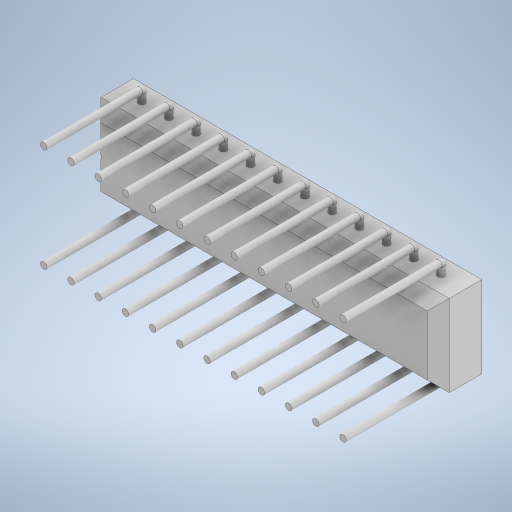
# Autodesk Inventor part: LM1040
Saved by Autodesk Inventor 2024 (Build 280153000, 153)
## iProperties
Created: 2023-12-15
Part Number: LM1040
Material: Generic
Document SubType Name: Sheet Metal
Designer: user
Density: 1 g/cm^3
Sheet Metal Rule: Default
Appearance: Default
Author: user
Autodesk Inventor part; units mm, degrees
sketch "Sketch1" plane through (0, 0, 0) normal (0, 0, 1) x (1, 0, 0)
  line L0 (0, 0) -> (32, 0)
  line L1 (32, 0) -> (32, 7.5)
  line L2 (32, 7.5) -> (0, 7.5)
  line L3 (0, 7.5) -> (0, 5)
  line L4 (0, 0) -> (0, 2.5)
  arc A0 (0, 2.5) -> (0, 5) centre (-0.2534, 3.75) ccw
  dimension "d0" = 32
  dimension "d1" = 7.5
  dimension "d2" = 2.5
  dimension "d3" = 2.5
  constraints: 10 end point, 2 point on circle, 2 vertical, 1 centre point, 1 horizontal, 1 parallel, 1 perpendicular
  measures "d0" distance of L2.end L1.end
  measures "d1" distance of L1.end L0.end
  measures "d2" distance of L2.end L3.end
  measures "d3" distance of L0.start L4.end
extrude "Extrusion1" add sketch "Sketch1" along normal blind 5
sketch "Sketch2" plane through (0, 7.5, 0) normal (0, 1, 0) x (1, 0, 0)
  line L0 (0, 0) -> (0, -5) projected
  circle A0 centre (29.75, -2.5) radius 0.3
  circle A1 centre (27.25, -2.5) radius 0.3
  circle A2 centre (24.75, -2.5) radius 0.3
  circle A3 centre (22.25, -2.5) radius 0.3
  circle A4 centre (19.75, -2.5) radius 0.3
  circle A5 centre (17.25, -2.5) radius 0.3
  circle A6 centre (14.75, -2.5) radius 0.3
  circle A7 centre (12.25, -2.5) radius 0.3
  circle A8 centre (9.75, -2.5) radius 0.3
  circle A9 centre (7.25, -2.5) radius 0.3
  circle A10 centre (4.75, -2.5) radius 0.3
  circle A11 centre (2.25, -2.5) radius 0.3
  line L1 (32, 0) -> (32, -5) projected
  line L2 (32, -2.5) -> (31.5682, -2.5)
  line L3 (0, -5) -> (32, -5) projected
  line L4 (32, -5) -> (29.75, -5)
  line L5 (29.75, -5) -> (27.25, -5)
  line L6 (27.25, -5) -> (24.75, -5)
  line L7 (24.75, -5) -> (22.25, -5)
  line L8 (22.25, -5) -> (19.75, -5)
  line L9 (19.75, -5) -> (17.25, -5)
  line L10 (17.25, -5) -> (14.75, -5)
  line L11 (14.75, -5) -> (12.25, -5)
  line L12 (12.25, -5) -> (9.75, -5)
  line L13 (9.75, -5) -> (7.25, -5)
  line L14 (7.25, -5) -> (4.75, -5)
  line L15 (4.75, -5) -> (2.25, -5)
  dimension "d8" = 0.6
  dimension "d10" = 0.6
  dimension "d21" = 0.6
  dimension "d22" = 0.6
  dimension "d23" = 0.6
  dimension "d24" = 0.6
  dimension "d25" = 0.6
  dimension "d26" = 0.6
  dimension "d27" = 0.6
  dimension "d28" = 0.6
  dimension "d29" = 0.6
  dimension "d30" = 0.6
  constraints: 26 end point, 12 centre point, 1 midpoint, 13 other
  measures "d8" diameter of A0
  measures "d10" diameter of A1
  measures "d21" diameter of A2
  measures "d22" diameter of A3
  measures "d23" diameter of A4
  measures "d24" diameter of A5
  measures "d25" diameter of A6
  measures "d26" diameter of A7
  measures "d27" diameter of A8
  measures "d28" diameter of A9
  measures "d29" diameter of A10
  measures "d30" diameter of A11
ref_plane "Work Plane1" through (29.75, 7.5, 5) normal (-1, 0, 0) x (0, -1, 0)
ref_plane "Work Plane2" through (27.25, 7.5, 5) normal (-1, 0, 0) x (0, -1, 0)
ref_plane "Work Plane3" through (24.75, 7.5, 5) normal (-1, 0, 0) x (0, -1, 0)
ref_plane "Work Plane4" through (22.25, 7.5, 5) normal (-1, 0, 0) x (0, -1, 0)
ref_plane "Work Plane5" through (19.75, 7.5, 5) normal (-1, 0, 0) x (0, -1, 0)
ref_plane "Work Plane6" through (17.25, 7.5, 5) normal (-1, 0, 0) x (0, -1, 0)
ref_plane "Work Plane7" through (14.75, 7.5, 5) normal (-1, 0, 0) x (0, -1, 0)
ref_plane "Work Plane8" through (12.25, 7.5, 5) normal (-1, 0, 0) x (0, -1, 0)
ref_plane "Work Plane9" through (9.75, 7.5, 5) normal (-1, 0, 0) x (0, -1, 0)
ref_plane "Work Plane10" through (7.25, 7.5, 5) normal (-1, 0, 0) x (0, -1, 0)
ref_plane "Work Plane11" through (4.75, 7.5, 5) normal (-1, 0, 0) x (0, -1, 0)
ref_plane "Work Plane12" through (2.25, 7.5, 5) normal (-1, 0, 0) x (0, -1, 0)
sketch "Sketch3" plane through (29.75, 7.5, 5) normal (-1, 0, 0) x (0, -1, 0)
  line L0 (0, -2.5) -> (-0.8, -2.5)
  line L1 (-1, -2.3) -> (-1, 6.5)
  arc A0 (-1, -2.3) -> (-0.8, -2.5) centre (-0.8, -2.3) ccw
  line L2 (0, -2.5) -> (7.5, -2.5)
  line L3 (7.5, -5) -> (7.5, 0) projected
  line L4 (7.5, -2.5) -> (8.3, -2.5)
  line L5 (8.5, -2.3) -> (8.5, 6.5)
  arc A1 (8.3, -2.5) -> (8.5, -2.3) centre (8.3, -2.3) ccw
  point P0 (0, -5)
  point P1 (-1, -2.5)
  point P2 (8.5, -2.5)
  dimension "d31" = 2.5
  dimension "d32" = 1
  dimension "d33" = 9
  dimension "d34" = 0.2
  dimension "d37" = 1
  dimension "d38" = 9
  dimension "d39" = 0.2
  constraints: 10 end point, 5 point on line, 4 point on circle, 4 tangent, 2 centre point, 2 perpendicular, 1 midpoint
  measures "d31" distance of point (0, -5) L0.start
  measures "d32" distance of L0.start point (-1, -2.5)
  measures "d33" distance of point (-1, -2.5) L1.end
  measures "d34" radius of A0
  measures "d37" distance of L2.end point (8.5, -2.5)
  measures "d38" distance of point (8.5, -2.5) L5.end
  measures "d39" radius of A1
sweep "Sweep1" add profiles "Sketch2" path "Sketch3" path curves L1 A0 L0 L2 L4 A1 L5 contours A0
sketch "Sketch4" plane through (27.25, 7.5, 5) normal (-1, 0, 0) x (0, -1, 0)
  line L0 (0, -2.5) -> (-0.8, -2.5)
  line L1 (-1, -2.3) -> (-1, 6.5)
  arc A0 (-1, -2.3) -> (-0.8, -2.5) centre (-0.8, -2.3) ccw
  line L2 (0, -2.5) -> (7.5, -2.5)
  line L3 (7.5, -2.5) -> (8.3, -2.5)
  line L4 (8.5, -2.3) -> (8.5, 6.5)
  arc A1 (8.3, -2.5) -> (8.5, -2.3) centre (8.3, -2.3) ccw
  point P0 (0, -5)
  point P1 (-1, -2.5)
  point P2 (8.5, -2.5)
  dimension "d40" = 2.5
  dimension "d41" = 1
  dimension "d42" = 9
  dimension "d43" = 0.2
  dimension "d44" = 1
  dimension "d45" = 9
  dimension "d46" = 0.2
  constraints: 10 end point, 5 point on line, 4 point on circle, 4 tangent, 2 centre point, 2 perpendicular
  measures "d40" distance of point (0, -5) L0.start
  measures "d41" distance of L0.start point (-1, -2.5)
  measures "d42" distance of point (-1, -2.5) L1.end
  measures "d43" radius of A0
  measures "d44" distance of L2.end point (8.5, -2.5)
  measures "d45" distance of point (8.5, -2.5) L4.end
  measures "d46" radius of A1
sketch "Sketch5" plane through (24.75, 7.5, 5) normal (-1, 0, 0) x (0, -1, 0)
  line L0 (0, -2.5) -> (-0.8, -2.5)
  line L1 (-1, -2.3) -> (-1, 6.5)
  arc A0 (-1, -2.3) -> (-0.8, -2.5) centre (-0.8, -2.3) ccw
  line L2 (0, -2.5) -> (7.5, -2.5)
  line L3 (7.5, -2.5) -> (8.3, -2.5)
  line L4 (8.5, -2.3) -> (8.5, 6.5)
  arc A1 (8.3, -2.5) -> (8.5, -2.3) centre (8.3, -2.3) ccw
  point P0 (0, -5)
  point P1 (-1, -2.5)
  point P2 (8.5, -2.5)
  dimension "d47" = 2.5
  dimension "d48" = 1
  dimension "d49" = 9
  dimension "d50" = 0.2
  dimension "d51" = 1
  dimension "d52" = 9
  dimension "d53" = 0.2
  constraints: 10 end point, 5 point on line, 4 point on circle, 4 tangent, 2 centre point, 2 perpendicular
  measures "d47" distance of point (0, -5) L0.start
  measures "d48" distance of L0.start point (-1, -2.5)
  measures "d49" distance of point (-1, -2.5) L1.end
  measures "d50" radius of A0
  measures "d51" distance of L2.end point (8.5, -2.5)
  measures "d52" distance of point (8.5, -2.5) L4.end
  measures "d53" radius of A1
sketch "Sketch6" plane through (22.25, 7.5, 5) normal (-1, 0, 0) x (0, -1, 0)
  line L0 (0, -2.5) -> (-0.8, -2.5)
  line L1 (-1, -2.3) -> (-1, 6.5)
  arc A0 (-1, -2.3) -> (-0.8, -2.5) centre (-0.8, -2.3) ccw
  line L2 (0, -2.5) -> (7.5, -2.5)
  line L3 (7.5, -2.5) -> (8.3, -2.5)
  line L4 (8.5, -2.3) -> (8.5, 6.5)
  arc A1 (8.3, -2.5) -> (8.5, -2.3) centre (8.3, -2.3) ccw
  point P0 (0, -5)
  point P1 (-1, -2.5)
  point P2 (8.5, -2.5)
  dimension "d54" = 2.5
  dimension "d55" = 1
  dimension "d56" = 9
  dimension "d57" = 0.2
  dimension "d58" = 1
  dimension "d59" = 9
  dimension "d60" = 0.2
  constraints: 10 end point, 5 point on line, 4 point on circle, 4 tangent, 2 centre point, 2 perpendicular
  measures "d54" distance of point (0, -5) L0.start
  measures "d55" distance of L0.start point (-1, -2.5)
  measures "d56" distance of point (-1, -2.5) L1.end
  measures "d57" radius of A0
  measures "d58" distance of L2.end point (8.5, -2.5)
  measures "d59" distance of point (8.5, -2.5) L4.end
  measures "d60" radius of A1
sketch "Sketch7" plane through (19.75, 7.5, 5) normal (-1, 0, 0) x (0, -1, 0)
  line L0 (0, -2.5) -> (-0.8, -2.5)
  line L1 (-1, -2.3) -> (-1, 6.5)
  arc A0 (-1, -2.3) -> (-0.8, -2.5) centre (-0.8, -2.3) ccw
  line L2 (0, -2.5) -> (7.5, -2.5)
  line L3 (7.5, -2.5) -> (8.3, -2.5)
  line L4 (8.5, -2.3) -> (8.5, 6.5)
  arc A1 (8.3, -2.5) -> (8.5, -2.3) centre (8.3, -2.3) ccw
  point P0 (0, -5)
  point P1 (-1, -2.5)
  point P2 (8.5, -2.5)
  dimension "d61" = 2.5
  dimension "d62" = 1
  dimension "d63" = 9
  dimension "d64" = 0.2
  dimension "d65" = 1
  dimension "d66" = 9
  dimension "d67" = 0.2
  constraints: 10 end point, 5 point on line, 4 point on circle, 4 tangent, 2 centre point, 2 perpendicular
  measures "d61" distance of point (0, -5) L0.start
  measures "d62" distance of L0.start point (-1, -2.5)
  measures "d63" distance of point (-1, -2.5) L1.end
  measures "d64" radius of A0
  measures "d65" distance of L2.end point (8.5, -2.5)
  measures "d66" distance of point (8.5, -2.5) L4.end
  measures "d67" radius of A1
sketch "Sketch8" plane through (17.25, 7.5, 5) normal (-1, 0, 0) x (0, -1, 0)
  line L0 (0, -2.5) -> (-0.8, -2.5)
  line L1 (-1, -2.3) -> (-1, 6.5)
  arc A0 (-1, -2.3) -> (-0.8, -2.5) centre (-0.8, -2.3) ccw
  line L2 (0, -2.5) -> (7.5, -2.5)
  line L3 (7.5, -2.5) -> (8.3, -2.5)
  line L4 (8.5, -2.3) -> (8.5, 6.5)
  arc A1 (8.3, -2.5) -> (8.5, -2.3) centre (8.3, -2.3) ccw
  point P0 (0, -5)
  point P1 (-1, -2.5)
  point P2 (8.5, -2.5)
  dimension "d68" = 2.5
  dimension "d69" = 1
  dimension "d70" = 9
  dimension "d71" = 0.2
  dimension "d72" = 1
  dimension "d73" = 9
  dimension "d74" = 0.2
  constraints: 10 end point, 5 point on line, 4 point on circle, 4 tangent, 2 centre point, 2 perpendicular
  measures "d68" distance of point (0, -5) L0.start
  measures "d69" distance of L0.start point (-1, -2.5)
  measures "d70" distance of point (-1, -2.5) L1.end
  measures "d71" radius of A0
  measures "d72" distance of L2.end point (8.5, -2.5)
  measures "d73" distance of point (8.5, -2.5) L4.end
  measures "d74" radius of A1
sketch "Sketch9" plane through (14.75, 7.5, 5) normal (-1, 0, 0) x (0, -1, 0)
  line L0 (0, -2.5) -> (-0.8, -2.5)
  line L1 (-1, -2.3) -> (-1, 6.5)
  arc A0 (-1, -2.3) -> (-0.8, -2.5) centre (-0.8, -2.3) ccw
  line L2 (0, -2.5) -> (7.5, -2.5)
  line L3 (7.5, -2.5) -> (8.3, -2.5)
  line L4 (8.5, -2.3) -> (8.5, 6.5)
  arc A1 (8.3, -2.5) -> (8.5, -2.3) centre (8.3, -2.3) ccw
  point P0 (0, -5)
  point P1 (-1, -2.5)
  point P2 (8.5, -2.5)
  dimension "d75" = 2.5
  dimension "d76" = 1
  dimension "d77" = 9
  dimension "d78" = 0.2
  dimension "d79" = 1
  dimension "d80" = 9
  dimension "d81" = 0.2
  constraints: 10 end point, 5 point on line, 4 point on circle, 4 tangent, 2 centre point, 2 perpendicular
  measures "d75" distance of point (0, -5) L0.start
  measures "d76" distance of L0.start point (-1, -2.5)
  measures "d77" distance of point (-1, -2.5) L1.end
  measures "d78" radius of A0
  measures "d79" distance of L2.end point (8.5, -2.5)
  measures "d80" distance of point (8.5, -2.5) L4.end
  measures "d81" radius of A1
sketch "Sketch10" plane through (12.25, 7.5, 5) normal (-1, 0, 0) x (0, -1, 0)
  line L0 (0, -2.5) -> (-0.8, -2.5)
  line L1 (-1, -2.3) -> (-1, 6.5)
  arc A0 (-1, -2.3) -> (-0.8, -2.5) centre (-0.8, -2.3) ccw
  line L2 (0, -2.5) -> (7.5, -2.5)
  line L3 (7.5, -2.5) -> (8.3, -2.5)
  line L4 (8.5, -2.3) -> (8.5, 6.5)
  arc A1 (8.3, -2.5) -> (8.5, -2.3) centre (8.3, -2.3) ccw
  point P0 (0, -5)
  point P1 (-1, -2.5)
  point P2 (8.5, -2.5)
  dimension "d82" = 2.5
  dimension "d83" = 1
  dimension "d84" = 9
  dimension "d85" = 0.2
  dimension "d86" = 1
  dimension "d87" = 9
  dimension "d88" = 0.2
  constraints: 10 end point, 5 point on line, 4 point on circle, 4 tangent, 2 centre point, 2 perpendicular
  measures "d82" distance of point (0, -5) L0.start
  measures "d83" distance of L0.start point (-1, -2.5)
  measures "d84" distance of point (-1, -2.5) L1.end
  measures "d85" radius of A0
  measures "d86" distance of L2.end point (8.5, -2.5)
  measures "d87" distance of point (8.5, -2.5) L4.end
  measures "d88" radius of A1
sketch "Sketch11" plane through (9.75, 7.5, 5) normal (-1, 0, 0) x (0, -1, 0)
  line L0 (0, -2.5) -> (-0.8, -2.5)
  line L1 (-1, -2.3) -> (-1, 6.5)
  arc A0 (-1, -2.3) -> (-0.8, -2.5) centre (-0.8, -2.3) ccw
  line L2 (0, -2.5) -> (7.5, -2.5)
  line L3 (7.5, -2.5) -> (8.3, -2.5)
  line L4 (8.5, -2.3) -> (8.5, 6.5)
  arc A1 (8.3, -2.5) -> (8.5, -2.3) centre (8.3, -2.3) ccw
  point P0 (0, -5)
  point P1 (-1, -2.5)
  point P2 (8.5, -2.5)
  dimension "d89" = 2.5
  dimension "d90" = 1
  dimension "d91" = 9
  dimension "d92" = 0.2
  dimension "d93" = 1
  dimension "d94" = 9
  dimension "d95" = 0.2
  constraints: 10 end point, 5 point on line, 4 point on circle, 4 tangent, 2 centre point, 2 perpendicular
  measures "d89" distance of point (0, -5) L0.start
  measures "d90" distance of L0.start point (-1, -2.5)
  measures "d91" distance of point (-1, -2.5) L1.end
  measures "d92" radius of A0
  measures "d93" distance of L2.end point (8.5, -2.5)
  measures "d94" distance of point (8.5, -2.5) L4.end
  measures "d95" radius of A1
sketch "Sketch12" plane through (7.25, 7.5, 5) normal (-1, 0, 0) x (0, -1, 0)
  line L0 (0, -2.5) -> (-0.8, -2.5)
  line L1 (-1, -2.3) -> (-1, 6.5)
  arc A0 (-1, -2.3) -> (-0.8, -2.5) centre (-0.8, -2.3) ccw
  line L2 (0, -2.5) -> (7.5, -2.5)
  line L3 (7.5, -2.5) -> (8.3, -2.5)
  line L4 (8.5, -2.3) -> (8.5, 6.5)
  arc A1 (8.3, -2.5) -> (8.5, -2.3) centre (8.3, -2.3) ccw
  point P0 (0, -5)
  point P1 (-1, -2.5)
  point P2 (8.5, -2.5)
  dimension "d96" = 2.5
  dimension "d97" = 1
  dimension "d98" = 9
  dimension "d99" = 0.2
  dimension "d100" = 1
  dimension "d101" = 9
  dimension "d102" = 0.2
  constraints: 10 end point, 5 point on line, 4 point on circle, 4 tangent, 2 centre point, 2 perpendicular
  measures "d96" distance of point (0, -5) L0.start
  measures "d97" distance of L0.start point (-1, -2.5)
  measures "d98" distance of point (-1, -2.5) L1.end
  measures "d99" radius of A0
  measures "d100" distance of L2.end point (8.5, -2.5)
  measures "d101" distance of point (8.5, -2.5) L4.end
  measures "d102" radius of A1
sketch "Sketch13" plane through (4.75, 7.5, 5) normal (-1, 0, 0) x (0, -1, 0)
  line L0 (0, -2.5) -> (-0.8, -2.5)
  line L1 (-1, -2.3) -> (-1, 6.5)
  arc A0 (-1, -2.3) -> (-0.8, -2.5) centre (-0.8, -2.3) ccw
  line L2 (0, -2.5) -> (7.5, -2.5)
  line L3 (7.5, -2.5) -> (8.3, -2.5)
  line L4 (8.5, -2.3) -> (8.5, 6.5)
  arc A1 (8.3, -2.5) -> (8.5, -2.3) centre (8.3, -2.3) ccw
  point P0 (0, -5)
  point P1 (-1, -2.5)
  point P2 (8.5, -2.5)
  dimension "d103" = 2.5
  dimension "d104" = 1
  dimension "d105" = 9
  dimension "d106" = 0.2
  dimension "d107" = 1
  dimension "d108" = 9
  dimension "d109" = 0.2
  constraints: 10 end point, 5 point on line, 4 point on circle, 4 tangent, 2 centre point, 2 perpendicular
  measures "d103" distance of point (0, -5) L0.start
  measures "d104" distance of L0.start point (-1, -2.5)
  measures "d105" distance of point (-1, -2.5) L1.end
  measures "d106" radius of A0
  measures "d107" distance of L2.end point (8.5, -2.5)
  measures "d108" distance of point (8.5, -2.5) L4.end
  measures "d109" radius of A1
sketch "Sketch14" plane through (2.25, 7.5, 5) normal (-1, 0, 0) x (0, -1, 0)
  line L0 (0, -2.5) -> (-0.8, -2.5)
  line L1 (-1, -2.3) -> (-1, 6.5)
  arc A0 (-1, -2.3) -> (-0.8, -2.5) centre (-0.8, -2.3) ccw
  line L2 (0, -2.5) -> (7.5, -2.5)
  line L3 (7.5, -2.5) -> (8.3, -2.5)
  line L4 (8.5, -2.3) -> (8.5, 6.5)
  arc A1 (8.3, -2.5) -> (8.5, -2.3) centre (8.3, -2.3) ccw
  point P0 (0, -5)
  point P1 (-1, -2.5)
  point P2 (8.5, -2.5)
  dimension "d110" = 2.5
  dimension "d111" = 1
  dimension "d112" = 9
  dimension "d113" = 0.2
  dimension "d114" = 1
  dimension "d115" = 9
  dimension "d116" = 0.2
  constraints: 10 end point, 5 point on line, 4 point on circle, 4 tangent, 2 centre point, 2 perpendicular
  measures "d110" distance of point (0, -5) L0.start
  measures "d111" distance of L0.start point (-1, -2.5)
  measures "d112" distance of point (-1, -2.5) L1.end
  measures "d113" radius of A0
  measures "d114" distance of L2.end point (8.5, -2.5)
  measures "d115" distance of point (8.5, -2.5) L4.end
  measures "d116" radius of A1
sketch "Sketch15" plane through (29.75, 7.5, 5) normal (-1, 0, 0) x (0, -1, 0)
  line L0 (0, -2.5) -> (-0.8, -2.5)
  line L1 (-1, -2.3) -> (-1, 6.5)
  arc A0 (-1, -2.3) -> (-0.8, -2.5) centre (-0.8, -2.3) ccw
  line L2 (0, -2.5) -> (7.5, -2.5)
  line L3 (7.5, -2.5) -> (8.3, -2.5)
  line L4 (8.5, -2.3) -> (8.5, 6.5)
  arc A1 (8.3, -2.5) -> (8.5, -2.3) centre (8.3, -2.3) ccw
  point P0 (0, -5)
  point P1 (-1, -2.5)
  point P2 (8.5, -2.5)
  dimension "d117" = 2.5
  dimension "d118" = 1
  dimension "d119" = 9
  dimension "d120" = 0.2
  dimension "d121" = 1
  dimension "d122" = 9
  dimension "d123" = 0.2
  constraints: 10 end point, 5 point on line, 4 point on circle, 4 tangent, 2 centre point, 2 perpendicular
  measures "d117" distance of point (0, -5) L0.start
  measures "d118" distance of L0.start point (-1, -2.5)
  measures "d119" distance of point (-1, -2.5) L1.end
  measures "d120" radius of A0
  measures "d121" distance of L2.end point (8.5, -2.5)
  measures "d122" distance of point (8.5, -2.5) L4.end
  measures "d123" radius of A1
sweep "Sweep2" add profiles "Sketch2" path "Sketch4" contours A1
sweep "Sweep3" add profiles "Sketch2" path "Sketch5" contours A2
sweep "Sweep4" add profiles "Sketch2" path "Sketch6" contours A3
sweep "Sweep5" add profiles "Sketch2" path "Sketch7" contours A4
sweep "Sweep6" add profiles "Sketch2" path "Sketch8" contours A5
sweep "Sweep7" add profiles "Sketch2" path "Sketch9" contours A6
sweep "Sweep8" add profiles "Sketch2" path "Sketch10" contours A7
sweep "Sweep9" add profiles "Sketch2" path "Sketch11" contours A8
sweep "Sweep10" add profiles "Sketch2" path "Sketch12" contours A9
sweep "Sweep11" add profiles "Sketch2" path "Sketch13" contours A10
sweep "Sweep12" add profiles "Sketch2" path "Sketch14" contours A11
chamfer "Chamfer1" distance 1 angle 45 2 edges at (16, 0, 0) (16, 7.5, 0)
chamfer "Chamfer2" distance 1 angle 45 1 edges at (32, 3.75, 0)
chamfer "Chamfer3" distance 1 angle 45 2 edges at (0, 1.75, 0) (0, 5.75, 0)
chamfer "Chamfer4" distance 1 angle 45 5 edges at (32, 3.75, 5) (16, 7.5, 5) (16, 0, 5) (0, 6.25, 5) (0, 1.25, 5)
sketch "Sketch16" plane through (0, 0, 0) normal (0, 0, -1) x (-1, 0, 0)
  line L0 (-19.6607, 4.4201) -> (-12.5424, 4.4201) construction
  line L1 (-12.5424, 4.4201) -> (-12.5424, 2.8581) construction
  line L2 (-12.5424, 2.8581) -> (-19.6607, 2.8581) construction
  line L3 (-19.6607, 2.8581) -> (-19.6607, 4.4201) construction
  point P0 (0, 0)
  constraints: 2 other
equation "\"BendRadius\" = Thickness"
equation "\"BendReliefWidth\" = Thickness"
equation "\"BendReliefDepth\" = 0.5 * Thickness"
equation "\"CornerReliefSize\" = 4 * Thickness"
equation "\"MinimumRemnant\" = 2 * Thickness"
equation "\"TransitionRadius\" = BendRadius"
equation "\"JacobiRadiusSize\" = BendRadius"
equation "\"GapSize\" = Thickness"
equation "\"Thickness\" = 3.048"
body "Solid1"
